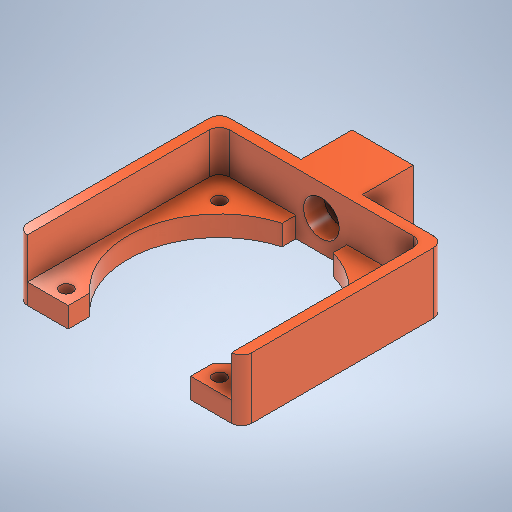
# Autodesk Inventor part: CameraMount1
Saved by Autodesk Inventor 2025 (Build 290162010, 162A)
## iProperties
Created: 2024-07-04
Part Number: CameraMount1
Material: Generic
Document SubType Name: Modeling
Designer: rolan
Density: 1 g/cm^3
Appearance: Default
Author: rolan
Autodesk Inventor part; units mm, degrees
ref_plane "YZ Plane" through (0, 0, 0) normal (1, 0, 0) x (0, 1, 0)
ref_plane "XZ Plane" through (0, 0, 0) normal (0, 1, 0) x (-1, 0, 0)
ref_plane "XY Plane" through (0, 0, 0) normal (0, 0, 1) x (1, 0, 0)
sketch "Sketch1" plane through (0, 0, 0) normal (0, 1, 0) x (-1, 0, 0)
  line L0 (19, 19) -> (-19, 19) construction
  line L1 (-19, 19) -> (-19, -19) construction
  line L2 (-19, -19) -> (19, -19) construction
  line L3 (19, -19) -> (19, 19) construction
  line L4 (19, 19) -> (-19, -19) construction
  line L5 (-19, 19) -> (19, -19) construction
  circle A0 centre (15, -15) radius 1.25
  circle A1 centre (-15, -15) radius 1.25
  circle A2 centre (-15, 15) radius 1.25
  circle A3 centre (15, 15) radius 1.25
  line L6 (-20, 20) -> (-20, -20)
  line L7 (-20, -20) -> (20, -20)
  line L8 (20, -20) -> (20, 20)
  line L9 (20, 20) -> (-20, -20) construction
  line L10 (-20, 20) -> (20, -20) construction
  line L11 (-22, 22) -> (-22, -22)
  line L12 (-22, -22) -> (22, -22)
  line L13 (22, -22) -> (22, 22)
  line L14 (22, 22) -> (-22, -22) construction
  line L15 (-22, 22) -> (22, -22) construction
  line L16 (12, 13.4164) -> (12, 22)
  line L17 (-12, 13.4164) -> (-12, 22)
  line L18 (20, 20) -> (12, 20)
  line L19 (-12, 20) -> (-20, 20)
  line L20 (22, 22) -> (12, 22)
  line L21 (-12, 22) -> (-22, 22)
  line L22 (5, -17.2916) -> (5, -20)
  line L23 (-5, -20) -> (-5, -17.2916)
  arc A4 (-12, 13.4164) -> (-5, -17.2916) centre (0, 0) ccw
  arc A5 (5, -17.2916) -> (12, 13.4164) centre (0, 0) ccw
  dimension "d0" = 38
  dimension "d1" = 38
  dimension "d2" = 4
  dimension "d3" = 4
  dimension "d4" = 4
  dimension "d5" = 4
  dimension "d6" = 2.5
  dimension "d7" = 2.5
  dimension "d8" = 2.5
  dimension "d9" = 2.5
  dimension "d11" = 40
  dimension "d12" = 40
  dimension "d13" = 44
  dimension "d14" = 44
  dimension "d15" = 10
  dimension "d16" = 10
  dimension "d17" = 17
  dimension "d18" = 17
  dimension "d19" = 18
  dimension "d20" = 18
  constraints: 48 end point, 10 perpendicular, 9 parallel, 6 centre point, 6 midpoint, 5 horizontal, 4 point on circle, 4 point on line, 2 horizontal alignment, 2 vertical alignment, 1 coincident
  measures "d0" distance of L1.end L2.end
  measures "d1" distance of L0.end L1.end
  measures "d2" distance from line of L2 A0.centre
  measures "d3" distance from line of L3 A0.centre
  measures "d4" distance from line of L0 A2.centre
  measures "d5" distance from line of L1 A2.centre
  measures "d6" diameter of A0
  measures "d7" diameter of A1
  measures "d8" diameter of A2
  measures "d9" diameter of A3
  measures "d11" distance of L7.end L6.end
  measures "d12" distance of L6.end L6.start
  measures "d13" distance of L12.end L11.end
  measures "d14" distance of L11.end L11.start
  measures "d15" distance from line of L13 L16.end
  measures "d16" distance from line of L11.start L17
  measures "d17" distance between parallel lines of L11 L23
  measures "d18" distance between parallel lines of L13 L22
  measures "d19" radius of A4
  measures "d20" radius of A5
extrude "Extrusion1" add sketch "Sketch1" along normal blind 4
sketch "Sketch2" plane through (0, 4, 0) normal (0, 1, 0) x (1, 0, 0)
  line L0 (22, 22) -> (-22, 22) projected
  line L1 (-22, 22) -> (22, 22)
  line L2 (12, -22) -> (22, -22) projected
  line L3 (22, 22) -> (22, -22)
  line L4 (22, -22) -> (12, -22)
  line L5 (12, -22) -> (12, -20)
  line L6 (12, -20) -> (20, -20)
  line L7 (20, -20) -> (20, 20)
  line L8 (20, 20) -> (-20, 20)
  line L9 (-20, 20) -> (-20, -20)
  line L10 (-22, -22) -> (-12, -22) projected
  line L11 (-20, 20) -> (20, 20) construction
  line L12 (-20, -20) -> (-12, -20)
  line L13 (-12, -20) -> (-12, -22)
  line L14 (-12, -22) -> (-22, -22)
  line L15 (-22, -22) -> (-22, 22)
  point P0 (0, 0)
  dimension "d23" = 2
  dimension "d24" = 8
  dimension "d25" = 40
  dimension "d26" = 40
  dimension "d27" = 40
  dimension "d28" = 90
  constraints: 26 end point, 10 perpendicular, 3 collinear, 1 horizontal
  measures "d23" distance of L2.start L5.end
  measures "d24" distance of L5.end L6.end
  measures "d25" distance of L6.end L7.end
  measures "d26" distance of L7.end L8.end
  measures "d27" distance of L8.end L9.end
  measures "d28" angle of L9 L11
extrude "Extrusion2" add sketch "Sketch2" along normal blind 8
sketch "Sketch3" plane through (0, 12, 0) normal (0, 1, 0) x (1, 0, 0)
  line L0 (-24.6321, -17.6536) -> (24.6321, -17.6536)
  line L1 (24.6321, -17.6536) -> (24.6321, -22.4819)
  line L2 (24.6321, -22.4819) -> (-24.6321, -22.4819)
  line L3 (-24.6321, -22.4819) -> (-24.6321, -17.6536)
  line L4 (-24.6321, -17.6536) -> (24.6321, -22.4819) construction
  line L5 (24.6321, -17.6536) -> (-24.6321, -22.4819) construction
  point P0 (0, 0)
  point P1 (0, -20.0678)
  constraints: 12 end point, 2 midpoint, 2 parallel, 1 horizontal, 1 perpendicular
extrude "Extrusion3" cut sketch "Sketch3" against normal through all
fillet "Fillet2" radius 2 6 edges at (20, 8, -20) (-20, 8, -20) (-22, 6, 17.6536) (22, 6, 17.6536) (22, 6, -22) (-22, 6, -22)
sketch "Sketch4" plane through (20, 0, -22) normal (0, 0, -1) x (-1, 0, 0)
  line L0 (0, 0) -> (40, 0) projected
  line L1 (26, 0) -> (14, 0)
  line L2 (14, 0) -> (14, 12)
  line L3 (14, 12) -> (26, 12)
  line L4 (26, 12) -> (26, 0)
  point P0 (20, 0)
  point P1 (20, 0)
  dimension "d35" = 12
  dimension "d36" = 12
  dimension "d37" = 6
  constraints: 8 end point, 2 parallel, 1 horizontal, 1 midpoint, 1 perpendicular, 1 point on line
  measures "d35" distance of L1.end L2.end
  measures "d36" distance of L1.end L1.start
  measures "d37" distance from line of L2 point (20, 0)
extrude "Extrusion4" add sketch "Sketch4" along normal blind 10
sketch "Sketch5" plane through (-5, 0, -20) normal (0, 0, 1) x (1, 0, 0)
  circle A0 centre (5, 6) radius 3.5
  line L0 (-13, 12) -> (23, 12) projected
  line L1 (27, 0) -> (27, 12) projected
  point P0 (5, 0)
  dimension "d40" = 7
  dimension "d41" = 6
  dimension "d42" = 22
  constraints: 1 centre point
  measures "d40" diameter of A0
  measures "d41" distance from line of L0 A0.centre
  measures "d42" distance from line of L1 A0.centre
extrude "Extrusion5" cut sketch "Sketch5" against normal blind 4
sketch "Sketch6" plane through (0, 6, -24) normal (0, 0, 1) x (1, 0, 0)
  circle A0 centre (0, 0) radius 2
  line L0 (-18, 6) -> (18, 6) projected
  line L1 (22, -6) -> (22, 6) projected
  point P0 (0, -6)
  dimension "d45" = 4
  dimension "d46" = 6
  dimension "d47" = 22
  constraints: 1 centre point
  measures "d45" diameter of A0
  measures "d46" distance from line of L0 A0.centre
  measures "d47" distance from line of L1 A0.centre
extrude "Extrusion6" cut sketch "Sketch6" against normal through all
body "Solid1"
